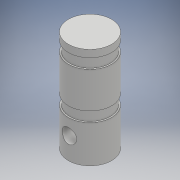
# Autodesk Inventor part: waleczek_do_sprezyn_fi6
Saved by Autodesk Inventor 2017 (Build 210142000, 142)
## iProperties
Created: 2021-05-20
Part Number: waleczek_do_sprezyn_fi6
Material: Generic
Document SubType Name: Modeling
Designer: majch
Density: 1 g/cm^3
Appearance: Default
Author: majch
Autodesk Inventor part; units mm, degrees
ref_plane "YZ Plane" through (0, 0, 0) normal (1, 0, 0) x (0, 1, 0)
ref_plane "XZ Plane" through (0, 0, 0) normal (0, 1, 0) x (-1, 0, 0)
ref_plane "XY Plane" through (0, 0, 0) normal (0, 0, 1) x (1, 0, 0)
sketch "Sketch2" plane through (0, 0, 0) normal (0, 1, 0) x (-1, 0, 0)
  line L0 (0, 15) -> (0, -17) construction
  line L1 (0, 15) -> (3, 15)
  line L2 (3, 15) -> (3, 14)
  line L3 (3, 14) -> (2.8, 14)
  line L4 (2.8, 14) -> (2.8, 12.6)
  line L5 (2.8, 12.6) -> (3, 12.6)
  line L6 (3, 12.6) -> (3, 7.6)
  line L7 (3, 7.6) -> (2.8, 7.6)
  line L8 (2.8, 7.6) -> (2.8, 6.2)
  line L9 (2.8, 6.2) -> (3, 6.2)
  line L10 (3, 6.2) -> (3, 1)
  line L11 (3, 1) -> (0, 1)
  line L12 (0, 15) -> (0, 1)
  point P0 (0, 0)
  dimension "d3" = 3
  dimension "d6" = 1
  dimension "d7" = 0.2
  dimension "d8" = 1.4
  dimension "d9" = 0.2
  dimension "d10" = 5
  dimension "d11" = 0.2
  dimension "d12" = 1.4
  dimension "d13" = 0.2
  dimension "d14" = 5.2
  dimension "d15" = 3
  constraints: 26 end point, 7 point on line, 2 perpendicular, 2 vertical, 1 collinear, 1 horizontal
  measures "d3" distance of L0.start L1.end
  measures "d6" distance of L1.end L2.end
  measures "d7" distance of L2.end L3.end
  measures "d8" distance of L3.end L4.end
  measures "d9" distance of L4.end L5.end
  measures "d10" distance of L5.end L6.end
  measures "d11" distance of L6.end L7.end
  measures "d12" distance of L7.end L8.end
  measures "d13" distance of L8.end L9.end
  measures "d14" distance of L9.end L10.end
  measures "d15" distance of L10.end L11.end
revolve "Revolution1" add sketch "Sketch2" angle 360 about axis through (0, 0, 15) along (0, 0, -1)
sketch "Sketch3" plane through (0, 0, 0) normal (0, 1, 0) x (-1, 0, 0)
  circle A0 centre (0, 4) radius 1
  line L0 (-3, 1) -> (3, 1) projected
  point P0 (0, 0)
  dimension "d17" = 2
  dimension "d18" = 3
  constraints: 1 centre point
  measures "d17" diameter of A0
  measures "d18" distance from line of L0 A0.centre
extrude "Extrusion2" cut sketch "Sketch3" along normal through all both and the other way through all
body "Solid2"
